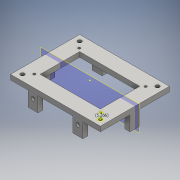
# Autodesk Inventor part: Joystickboard Holder
Saved by Autodesk Inventor 2016 SP2 (Build 200236200, 236)
## iProperties
Created: 2018-02-18
Part Number: Joystickboard Holder
Material: Generic
Document SubType Name: Modeling
Designer: Alexander
Density: 1 g/cm^3
Appearance: Default
Author: Alexander
Autodesk Inventor part; units mm, degrees
ref_plane "YZ Plane" through (0, 0, 0) normal (1, 0, 0) x (0, 1, 0)
ref_plane "XZ Plane" through (0, 0, 0) normal (0, 1, 0) x (-1, 0, 0)
ref_plane "XY Plane" through (0, 0, 0) normal (0, 0, 1) x (1, 0, 0)
sketch "Sketch1" plane through (0, 0, 0) normal (0, 0, 1) x (1, 0, 0)
  line L0 (-30.5, -20) -> (30.5, -20)
  line L1 (30.5, -20) -> (30.5, 20)
  line L2 (30.5, 20) -> (-30.5, 20)
  line L3 (-30.5, 20) -> (-30.5, -20)
  line L4 (-30.5, -20) -> (30.5, 20) construction
  line L5 (30.5, -20) -> (-30.5, 20) construction
  line L6 (-45.5, -35) -> (45.5, -35)
  line L7 (45.5, -35) -> (45.5, 35)
  line L8 (45.5, 35) -> (-45.5, 35)
  line L9 (-45.5, 35) -> (-45.5, -35)
  line L10 (-45.5, -35) -> (45.5, 35) construction
  line L11 (45.5, -35) -> (-45.5, 35) construction
  point P0 (0, 0)
  dimension "d0" = 61
  dimension "d1" = 40
  dimension "d2" = 15
  dimension "d3" = 15
  constraints: 24 end point, 4 midpoint, 4 parallel, 2 horizontal, 2 perpendicular
  measures "d0" distance of L1.end L2.end
  measures "d1" distance of L0.end L1.end
  measures "d2" distance between parallel lines of L8 L2
  measures "d3" distance between parallel lines of L7 L1
extrude "Rim" add sketch "Sketch1" along normal blind 5
sketch "Sketch2" plane through (0, 0, 5) normal (0, 0, 1) x (1, 0, 0)
  line L0 (-33.7, -22.765) -> (33.7, -22.765) construction
  line L1 (33.7, -22.765) -> (33.7, 22.765) construction
  line L2 (33.7, 22.765) -> (-33.7, 22.765) construction
  line L3 (-33.7, 22.765) -> (-33.7, -22.765) construction
  line L4 (-33.7, -22.765) -> (33.7, 22.765) construction
  line L5 (33.7, -22.765) -> (-33.7, 22.765) construction
  circle A0 centre (33.7, 22.765) radius 1.25
  line L6 (0, 22.765) -> (0, -22.765) construction
  line L7 (-30.5, -20) -> (-30.5, 20) projected
  line L8 (-30.5, 0) -> (33.7, 0) construction
  circle A1 centre (-33.7, 22.765) radius 1.25
  circle A2 centre (33.7, -22.765) radius 1.25
  circle A3 centre (-33.7, -22.765) radius 1.25
  point P0 (0, 0)
  dimension "d6" = 67.4
  dimension "d7" = 45.53
  dimension "d8" = 2.5
  constraints: 16 end point, 6 midpoint, 4 centre point, 3 symmetric about line, 2 parallel, 1 coincident, 1 horizontal, 1 perpendicular, 3 other
  measures "d6" distance of L1.end L2.end
  measures "d7" distance of L0.end L1.end
  measures "d8" diameter of A0
extrude "Pegs" cut sketch "Sketch2" against normal blind 3
sketch "Sketch3" plane through (0, 0, 0) normal (0, 0, -1) x (-1, 0, 0)
  line L0 (-39.5, 25.8246) -> (-42.25, 27.4123)
  line L1 (-36.75, 27.4123) -> (-39.5, 25.8246)
  line L2 (-42.25, 27.4123) -> (-42.25, 30.5877)
  line L3 (-36.75, 30.5877) -> (-36.75, 27.4123)
  circle A0 centre (-39.5, 29) radius 2
  line L4 (-39.5, 32.1754) -> (-36.75, 30.5877)
  line L5 (-42.25, 30.5877) -> (-39.5, 32.1754)
  line L6 (-45.5, 35) -> (35.9035, 35)
  line L7 (-45.5, 35) -> (-45.5, 29)
  line L8 (-45.5, -35) -> (-45.5, 35) projected
  line L9 (-45.5, 29) -> (-39.5, 29) construction
  line L10 (-45.5, -35) -> (-45.5, 35) projected
  line L11 (-45.5, 35) -> (45.5, 35) projected
  line L12 (0, 35) -> (0, -35) construction
  line L13 (45.5, -35) -> (-45.5, -35) projected
  line L14 (-45.5, 0) -> (45.5, 0) construction
  line L15 (45.5, 35) -> (45.5, -35) projected
  line L16 (39.5, 25.8246) -> (42.25, 27.4123)
  line L17 (36.75, 27.4123) -> (39.5, 25.8246)
  line L18 (42.25, 27.4123) -> (42.25, 30.5877)
  line L19 (36.75, 30.5877) -> (36.75, 27.4123)
  circle A1 centre (39.5, 29) radius 2
  line L20 (39.5, 32.1754) -> (36.75, 30.5877)
  line L21 (42.25, 30.5877) -> (39.5, 32.1754)
  line L22 (45.5, 29) -> (39.5, 29) construction
  line L23 (-39.5, -25.8246) -> (-42.25, -27.4123)
  line L24 (-36.75, -27.4123) -> (-39.5, -25.8246)
  line L25 (-42.25, -27.4123) -> (-42.25, -30.5877)
  line L26 (-36.75, -30.5877) -> (-36.75, -27.4123)
  circle A2 centre (-39.5, -29) radius 2
  line L27 (-39.5, -32.1754) -> (-36.75, -30.5877)
  line L28 (-42.25, -30.5877) -> (-39.5, -32.1754)
  line L29 (36.75, -30.5877) -> (36.75, -27.4123)
  line L30 (39.5, -32.1754) -> (36.75, -30.5877)
  circle A3 centre (39.5, -29) radius 2
  line L31 (42.25, -30.5877) -> (39.5, -32.1754)
  line L32 (42.25, -27.4123) -> (42.25, -30.5877)
  line L33 (39.5, -25.8246) -> (42.25, -27.4123)
  line L34 (36.75, -27.4123) -> (39.5, -25.8246)
  point P0 (0, 0)
  dimension "d11" = 3.1754
  dimension "d12" = 4
  dimension "d13" = 6
  dimension "d14" = 6
  constraints: 60 end point, 31 symmetric about line, 12 coincident, 4 centre point, 4 midpoint, 1 horizontal, 1 parallel, 1 perpendicular, 1 point on line, 16 other
  measures "d11" distance of L0.end L2.end
  measures "d12" diameter of A0
  measures "d13" distance of L6.start L7.end
  measures "d14" distance of L7.end L9.end
extrude "Nut Hexes" cut sketch "Sketch3" against normal blind 3 contours L0 L2 L5 L4 L3 L1 | L17 L19 L20 L21 L18 L16 | L24 L26 L27 L28 L25 L23 | L29 L34 L33 L32 L31 L30
sketch "Sketch4" plane through (0, 0, 0) normal (0, 0, -1) x (-1, 0, 0)
  circle A0 centre (-39.5, 29) radius 2 projected
  circle A1 centre (39.5, 29) radius 2 projected
  circle A2 centre (39.5, -29) radius 2 projected
  circle A3 centre (-39.5, -29) radius 2 projected
  point P0 (0, 0)
  constraints: 4 coincident
extrude "Bolt Holes" cut sketch "Sketch4" against normal up to next
sketch "For Construction" plane through (0, 0, 5) normal (0, 0, 1) x (1, 0, 0)
  circle A0 centre (33.7, -22.765) radius 1.25 projected
  circle A1 centre (39.5, -29) radius 2 projected
  point P0 (0, 0)
  point P1 (34.95, -22.765)
  point P2 (37.901, -27.7986)
  dimension "d19" = 5.2656
  constraints: 1 horizontal alignment, 3 other
sketch "Sketch7" plane through (0, 0, 0) normal (0, 0, -1) x (-1, 0, 0)
  line L0 (45.5, -35) -> (-45.5, -35) projected
  line L1 (45.5, -35) -> (0, -35)
  line L2 (27.75, -35) -> (17.75, -35)
  line L3 (17.75, -35) -> (17.75, -30)
  line L4 (17.75, -30) -> (27.75, -30)
  line L5 (27.75, -30) -> (27.75, -35)
  line L6 (0, -35) -> (0, 35.2559) construction
  line L7 (-27.75, -35) -> (-17.75, -35)
  line L8 (-17.75, -35) -> (-17.75, -30)
  line L9 (-17.75, -30) -> (-27.75, -30)
  line L10 (-27.75, -30) -> (-27.75, -35)
  point P0 (0, 0)
  point P1 (22.75, -35)
  point P2 (-22.75, -35)
  dimension "d20" = 5
  dimension "d21" = 10
  constraints: 20 end point, 5 symmetric about line, 3 midpoint, 2 parallel, 1 collinear, 1 horizontal, 1 perpendicular, 1 vertical
  measures "d20" distance of L2.end L3.end
  measures "d21" distance of L3.end L4.end
extrude "Attachment Points" add sketch "Sketch7" along normal blind 10
sketch "Sketch9" plane through (-45.5, -35, 5) normal (0, -1, 0) x (1, 0, 0)
  circle A0 centre (22.75, -10) radius 2 projected
  circle A1 centre (68.25, -10) radius 2 projected
  point P0 (45.5, -5)
  point P1 (22.75, -8)
  point P2 (68.25, -8)
  constraints: 2 vertical alignment, 2 other
extrude "Connection Holes" cut sketch "Sketch9" against normal up to next
sketch "Sketch10" plane through (0, 0, 0) normal (0, 0, -1) x (-1, 0, 0)
  line L0 (45.5, 35) -> (45.5, -35) projected
  line L1 (-45.5, -35) -> (-45.5, 35) projected
  line L2 (-45.5, 35) -> (45.5, 35) projected
  line L3 (0, 35) -> (45.5, 35)
  line L4 (0, 35) -> (-45.5, 35)
  line L5 (45.5, -5) -> (40.5, -5)
  line L6 (40.5, -5) -> (40.5, 5)
  line L7 (40.5, 5) -> (45.5, 5)
  line L8 (45.5, 5) -> (45.5, -5)
  line L9 (17.75, -35) -> (-17.75, -35) projected
  line L10 (0, -35) -> (0, -19.876) construction
  line L11 (-45.5, 35) -> (-45.5, -35)
  line L12 (-45.5, -5) -> (-40.5, -5)
  line L13 (-40.5, -5) -> (-40.5, 5)
  line L14 (-40.5, 5) -> (-45.5, 5)
  line L15 (-45.5, 5) -> (-45.5, -5)
  line L16 (27.75, 35) -> (17.75, 35)
  line L17 (17.75, 35) -> (17.75, 30)
  line L18 (17.75, 30) -> (27.75, 30)
  line L19 (27.75, 30) -> (27.75, 35)
  line L20 (-27.75, 35) -> (-17.75, 35)
  line L21 (-17.75, 35) -> (-17.75, 30)
  line L22 (-17.75, 30) -> (-27.75, 30)
  line L23 (-27.75, 30) -> (-27.75, 35)
  point P0 (0, 0)
  point P1 (45.5, 0)
  point P2 (-45.5, 0)
  point P3 (22.75, 35)
  point P4 (-22.75, 35)
  point P5 (45.5, 0)
  point P6 (-45.5, 0)
  point P7 (-45.5, 0)
  dimension "d28" = 5
  dimension "d29" = 10
  dimension "d30" = 5
  dimension "d31" = 10
  constraints: 40 end point, 10 symmetric about line, 9 midpoint, 4 parallel, 3 horizontal, 2 perpendicular, 1 collinear, 1 vertical
  measures "d28" distance of L5.start L5.end
  measures "d29" distance of L5.end L6.end
  measures "d30" distance of L16.end L17.end
  measures "d31" distance of L17.end L18.end
extrude "Legs 1" add sketch "Sketch10" along normal blind 15
sketch "Sketch11" plane through (0, 0, -10) normal (0, 0, -1) x (-1, 0, 0)
  line L0 (27.75, -30) -> (27.75, -35) projected
  line L1 (27.75, -30) -> (17.75, -30) projected
  line L2 (27.75, -35) -> (17.75, -35)
  line L3 (17.75, -35) -> (17.75, -30)
  line L4 (17.75, -30) -> (27.75, -30)
  line L5 (27.75, -30) -> (27.75, -35)
  line L6 (-17.75, -35) -> (-17.75, -30) projected
  line L7 (-27.75, -30) -> (-27.75, -35) projected
  line L8 (-17.75, -35) -> (-27.75, -35)
  line L9 (-27.75, -35) -> (-27.75, -30)
  line L10 (-27.75, -30) -> (-17.75, -30)
  line L11 (-17.75, -30) -> (-17.75, -35)
  point P0 (0, 0)
  constraints: 16 end point, 4 parallel, 2 horizontal, 2 perpendicular
extrude "Extrusion9" add sketch "Sketch11" along normal blind 5
ref_plane "Work Plane2" through (-30.5, 0, 0) normal (0, 1, 0) x (1, 0, 0)
sketch "Sketch12" plane through (17.75, -30, 0) normal (0, 1, 0) x (1, 0, 0)
  line L0 (5, 1.8246) -> (2.25, 3.4123)
  line L1 (7.75, 3.4123) -> (5, 1.8246)
  line L2 (2.25, 3.4123) -> (2.25, 6.5877)
  line L3 (7.75, 6.5877) -> (7.75, 3.4123)
  line L4 (5, 8.1754) -> (7.75, 6.5877)
  line L5 (2.25, 6.5877) -> (5, 8.1754)
  circle A0 centre (5, 5) radius 2 projected
  line L6 (0, 0) -> (0, 15) projected
  line L7 (-40.5, 1.8246) -> (-43.25, 3.4123)
  line L8 (-37.75, 3.4123) -> (-40.5, 1.8246)
  line L9 (-43.25, 3.4123) -> (-43.25, 6.5877)
  line L10 (-37.75, 6.5877) -> (-37.75, 3.4123)
  line L11 (-40.5, 8.1754) -> (-37.75, 6.5877)
  line L12 (-43.25, 6.5877) -> (-40.5, 8.1754)
  circle A1 centre (-40.5, 5) radius 2 projected
  line L13 (-35.5, 0) -> (-35.5, 15) projected
  point P0 (-17.75, 0)
  point P1 (-5.2731, 15.8695)
  point P2 (-26.4318, 33.2663)
  dimension "d36" = 3.1754
  dimension "d38" = 3.1754
  constraints: 24 end point, 4 coincident, 2 parallel, 26 other
  measures "d36" distance of L0.end L2.end
  measures "d38" distance of L7.end L9.end
extrude "Extrusion10" cut sketch "Sketch12" against normal blind 3
body "Solid1"
